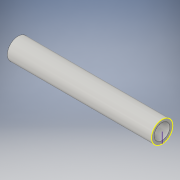
# Autodesk Inventor part: Pickup Pvc
Saved by Autodesk Inventor 2016 (Build 200138000, 138)
## iProperties
Created: 2015-11-25
Part Number: Pickup Pvc
Material: PVC-Piping
Document SubType Name: Modeling
Designer: Julia
Density: 1.4 g/cm^3
Appearance: Smooth - White
Author: Julia
Autodesk Inventor part; units mm, degrees
ref_plane "YZ Plane" through (0, 0, 0) normal (1, 0, 0) x (0, 1, 0)
ref_plane "XZ Plane" through (0, 0, 0) normal (0, 1, 0) x (-1, 0, 0)
ref_plane "XY Plane" through (0, 0, 0) normal (0, 0, 1) x (1, 0, 0)
sketch "Sketch1" plane through (0, 0, 0) normal (1, 0, 0) x (0, 1, 0)
  circle A0 centre (0, 0) radius 8.001
  dimension "d0" = 16.002
  constraints: 1 centre point, 1 coincident
  measures "d0" diameter of A0
extrude "Extrusion1" add sketch "Sketch1" along normal blind 107.95
sketch "Sketch2" plane through (107.95, 0, 0) normal (1, 0, 0) x (0, 0, -1)
  circle A0 centre (0, 0) radius 5.842
  dimension "d3" = 11.684
  constraints: 1 centre point, 1 coincident
  measures "d3" diameter of A0
extrude "Extrusion2" cut sketch "Sketch2" against normal blind 120.65
sketch "Sketch3" plane through (107.95, 0, 0) normal (1, 0, 0) x (0, 0, -1)
  line L0 (0, 0) -> (0, -8.001)
  circle A0 centre (0, 0) radius 8.001 projected
  line L1 (0, 0) -> (0, -8.001)
  line L2 (0, -8.001) -> (0, 0)
  constraints: 6 end point, 3 vertical, 1 vertical alignment, 1 other
body "Solid1"
